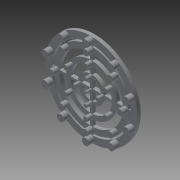
# Autodesk Inventor part: Cupholder cool2
Saved by Autodesk Inventor 2014 (Build 180170000, 170)
## iProperties
Created: 2014-07-17
Part Number: Cupholder cool2
Material: Generic
Document SubType Name: Modeling
Designer: quinn
Density: 1 g/cm^3
Appearance: Default
Author: quinn
Autodesk Inventor part; units mm, degrees
ref_plane "YZ Plane" through (0, 0, 0) normal (1, 0, 0) x (0, 1, 0)
ref_plane "XZ Plane" through (0, 0, 0) normal (0, 1, 0) x (-1, 0, 0)
ref_plane "XY Plane" through (0, 0, 0) normal (0, 0, 1) x (1, 0, 0)
sketch "Sketch1" plane through (0, 0, 0) normal (0, 0, 1) x (1, 0, 0)
  circle A0 centre (0, 38.1) radius 3.175
  circle A1 centre (0, 25.4) radius 2.54
  circle A2 centre (0, 12.7) radius 1.905
  circle A3 centre (0, 0) radius 1.27
  circle A4 centre (-26.9408, 26.9408) radius 3.175
  circle A5 centre (-38.1, 0) radius 3.175
  circle A6 centre (-26.9408, -26.9408) radius 3.175
  circle A7 centre (0, -38.1) radius 3.175
  circle A8 centre (26.9408, -26.9408) radius 3.175
  circle A9 centre (38.1, 0) radius 3.175
  circle A10 centre (26.9408, 26.9408) radius 3.175
  circle A11 centre (-21.997, 12.7) radius 2.54
  circle A12 centre (-21.997, -12.7) radius 2.54
  circle A13 centre (0, -25.4) radius 2.54
  circle A14 centre (21.997, -12.7) radius 2.54
  circle A15 centre (21.997, 12.7) radius 2.54
  circle A16 centre (-12.7, 0) radius 1.905
  circle A17 centre (0, -12.7) radius 1.905
  circle A18 centre (12.7, 0) radius 1.905
  circle A19 centre (0, 0) radius 43.18
  circle A20 centre (0, 0) radius 34.925
  circle A21 centre (0, 0) radius 41.275
  circle A22 centre (0, 0) radius 22.86
  circle A23 centre (0, 0) radius 27.94
  circle A24 centre (0, 0) radius 10.795
  circle A25 centre (0, 0) radius 14.605
  line L0 (-1.27, 0) -> (1.27, 0)
  line L1 (1.27, 0) -> (1.27, 50.7841)
  line L2 (1.27, 50.7841) -> (-1.27, 50.7841)
  line L3 (-1.27, 50.7841) -> (-1.27, 0)
  line L4 (-1.27, 0) -> (1.27, 0)
  line L5 (1.27, 0) -> (1.27, -50.7841)
  line L6 (1.27, -50.7841) -> (-1.27, -50.7841)
  line L7 (-1.27, -50.7841) -> (-1.27, 0)
  line L8 (0, 1.27) -> (50.7841, 1.27)
  line L9 (50.7841, 1.27) -> (50.7841, -1.27)
  line L10 (50.7841, -1.27) -> (0, -1.27)
  line L11 (0, -1.27) -> (0, 1.27)
  line L12 (0, 1.27) -> (-50.7841, 1.27)
  line L13 (-50.7841, 1.27) -> (-50.7841, -1.27)
  line L14 (-50.7841, -1.27) -> (0, -1.27)
  line L15 (0, -1.27) -> (0, 1.27)
  circle A26 centre (0, 0) radius 50.8
  dimension "d1" = 6.35
  dimension "d3" = 5.08
  dimension "d4" = 3.81
  dimension "d5" = 2.54
  dimension "d6" = 12.7
  dimension "d7" = 12.7
  dimension "d8" = 12.7
  dimension "d11" = 360
  dimension "d15" = 360
  dimension "d19" = 360
  dimension "d23" = 86.36
  dimension "d24" = 82.55
  dimension "d25" = 55.88
  dimension "d26" = 29.21
  dimension "d27" = 2.54
  dimension "d28" = 2.54
  dimension "d29" = 2.54
  dimension "d30" = 2.54
  dimension "d43" = 101.6
  constraints: 32 end point, 27 centre point, 8 coincident, 8 parallel, 4 horizontal, 4 perpendicular, 3 tangent, 2 point on circle, 39 other
  measures "d1" diameter of A0
  measures "d3" diameter of A1
  measures "d4" diameter of A2
  measures "d5" diameter of A3
  measures "d6" distance of A1.centre A0.centre
  measures "d7" distance of A2.centre A1.centre
  measures "d8" distance of point (0, 0) A2.centre
  measures "d23" diameter of A19
  measures "d24" diameter of A21
  measures "d25" diameter of A23
  measures "d26" diameter of A25
  measures "d27" distance of L2.end L1.end
  measures "d28" distance of L5.end L6.end
  measures "d29" distance of L8.end L9.end
  measures "d30" distance of L13.end L12.end
  measures "d43" diameter of A26
extrude "Extrusion1" add sketch "Sketch1" along normal blind 6.35 contours A0 L1 | L1 A0 L3 | L3 A0 | A10 | A4 | A15 | A1 L1 L3 | A1 L1 | A9 L10 L8 | L8 A9 | A11 | L3 A1 | A5 L12 L14 | A5 L12 | A9 L10 | L14 A5 | A8 | A6 | A12 | A14 | A18 L10 L8 | L8 A18 | A2 L1 L3 | A2 L1 | A7 L7 L5 | A7 L7 | L5 A7 | A16 L12 L14 | A16 L12 | L3 A2 | A18 L10 | A13 L7 L5 | A13 L7 | L14 A16 | L5 A13 | A17 L7 L5 | A17 L7 | L5 A17 | L0 L11 A3 | A3 L11 L0 | L11 L0 A3 | L0 L11 A3
extrude "Extrusion2" add sketch "Sketch1" against normal blind 3.81 contours A0 L1 | L1 A0 L3 | L3 A0 | A10 | A4 | A15 | A1 L1 L3 | A1 L1 | A9 L10 L8 | L8 A9 | A11 | L3 A1 | A5 L12 L14 | A5 L12 | A9 L10 | L14 A5 | A8 | A6 | A12 | A14 | A18 L10 L8 | L8 A18 | A7 L7 L5 | A7 L7 | L5 A7 | A16 L12 L14 | A16 L12 | A18 L10 | A13 L7 L5 | A13 L7 | L14 A16 | L5 A13 | A17 L7 L5 | A17 L7 | L5 A17 | L0 L11 A3 | A3 L11 L0 | L11 L0 A3 | L0 L11 A3
extrude "Extrusion3" add sketch "Sketch1" against normal blind 3.81 contours A0 L1 A21 A10 A20 | A0 A21 L1 | L1 A20 A0 | A0 L3 A21 | A20 L3 A0 | A0 L3 A20 A4 A21 | A21 L8 A9 A20 A10 | A4 A20 L12 A5 A21 | A21 A9 L8 | L8 A9 A20 | L12 A5 A21 | A21 L10 A9 | A20 A5 L12 | A9 L10 A20 | A5 L14 A21 | L10 A21 A8 A20 A9 | A20 L14 A5 | A5 L14 A20 A6 A21 | A21 L5 A7 A20 A8 | A6 A20 L7 A7 A21 | L7 A7 A21 | A21 A7 L5 | L5 A7 A20 | A20 A7 L7
extrude "Extrusion4" add sketch "Sketch1" against normal blind 3.81 contours L8 A18 A24 L1 A2 A25 | A25 A18 L8 | L1 A2 A25 | L12 A16 A25 | A25 L3 A2 A24 L12 A16 | A25 A2 L3 | A25 L10 A18 | L14 A16 A24 L7 A17 A25 | A25 A16 L14 | A25 L5 A17 A24 L10 A18 | A18 A24 L8 | L1 A24 A2 | L7 A17 A25 | L12 A24 A16 | A2 A24 L3 | A25 A17 L5 | L10 A24 A18 | A16 A24 L14 | L7 A24 A17 | A17 A24 L5
extrude "Extrusion5" add sketch "Sketch1" against normal blind 3.81 contours L1 A1 A23 | A23 A15 A22 L1 A1 | L3 A1 A22 A11 A23 | A23 A1 L3 | A23 L8 A22 A15 | A11 A22 L12 A23 | A23 L10 A22 L8 | L1 A22 A1 | L12 A22 L14 A23 | A1 A22 L3 | L14 A22 A12 A23 | A23 A14 A22 L10 | A12 A22 L7 A13 A23 | A23 L5 A13 A22 A14 | L7 A13 A23 | A23 A13 L5 | A22 A13 L7 | L5 A13 A22
extrude "Extrusion6" add sketch "Sketch1" against normal blind 3.81 contours A2 L1 L3 | A2 L1 | L3 A2
extrude "Extrusion7" add sketch "Sketch1" against normal blind 3.81 contours L1 A0 L3 | A0 A21 L1 | L1 A20 A0 | A21 L3 A19 L1 | A0 L3 A21 | A20 L3 A0 | A20 L1 A23 L3 | A19 L3 L2 L1 | L1 A1 A23 | L8 A19 L10 A21 | A21 A9 L8 | L8 L9 L10 A19 | A23 A1 L3 | L8 A9 A20 | A20 L10 A23 L8 | A1 L1 L3 | L12 A5 A21 | A21 L14 A19 L12 | A19 L14 L13 L12 | A9 L10 L8 | A21 L10 A9 | L12 A23 L14 A20 | A20 A5 L12 | A9 L10 A20 | A23 L10 A22 L8 | L1 A22 A1 | A5 L12 L14 | A5 L14 A21 | A20 L14 A5 | L12 A22 L14 A23 | A1 A22 L3 | A22 L10 A25 L8 | L1 A25 L3 A22 | L7 A21 L5 A19 | A19 L5 L6 L7 | L12 A25 L14 A22 | A25 A18 L8 | L1 A2 A25 | L7 A7 A21 | A21 A7 L5 | L12 A16 A25 | A25 A2 L3 | L5 A7 A20 | A20 L7 A23 L5 | A18 L10 L8 | A25 L10 A18 | A2 L1 L3 | A7 L7 L5 | A20 A7 L7 | L7 A13 A23 | A25 A16 L14 | A16 L12 L14 | A23 A13 L5 | A18 A24 L8 | L1 A24 A2 | L7 A25 L5 A22 | A22 A13 L7 | A13 L7 L5 | L7 A17 A25 | L12 A24 A16 | A2 A24 L3 | L5 A13 A22 | A25 A17 L5 | L10 A24 A18 | A24 L10 L5 L1 L8 | A24 L1 L8 L12 L3 | A17 L7 L5 | A16 A24 L14 | A24 L12 L3 L7 L14 | L1 A3 L8 | L7 A24 A17 | L12 A3 L3 | A17 A24 L5 | A24 L7 L14 L10 L5 | L10 A3 L5 | L0 L11 A3 | A3 L11 L0 | L11 L0 A3 | L7 A3 L14 | L0 L11 A3
extrude "Extrusion8" add sketch "Sketch1" against normal blind 3.81 contours L1 A26 L8 A19 | A19 L12 A26 L3 | L2 A26 | A26 L9 | A19 L7 A26 L14 | L13 A26 | L10 A26 L5 A19 | A26 L6
sketch "Sketch2" plane through (0, 0, 0) normal (0, 0, 1) x (1, 0, 0)
  circle A0 centre (0, 0) radius 50.8 projected
  circle A1 centre (0, 46.99) radius 3.81
  dimension "d46" = 7.62
  constraints: 1 centre point, 1 tangent
  measures "d46" diameter of A1
extrude "Extrusion9" add sketch "Sketch2" along normal blind 6.35 contours A1
pattern_circular "Circular Pattern1" count 10 over 360 about axis through (0, 0, 0) along (0, 0, 1) of "Extrusion9"
body "Solid1"
